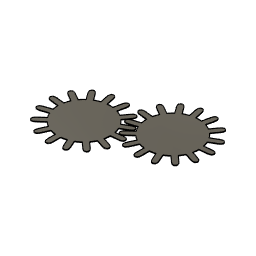
Gears (Autodesk Fusion 360 design; units mm, degrees)
Autodesk Fusion 360 part; units mm, degrees
sketch "Sketch1" plane through (0, 0, 0) normal (0, 0, 1) x (1, 0, 0)
  line L0 (-5, -63.7603) -> (-5, -49.7494)
  spline S0 degree 5 poles (-5, -63.7603) (-5, -64.7116) (-4.9363, -66.4553) (-4.6499, -68.5942) (-3.9278, -70.5592) (-2.6801, -71.8795) (-1.3088, -72.4515) (0, -72.5944) (1.3088, -72.4515) (2.68, -71.8795) (3.9278, -70.5592) (4.6499, -68.5942) (4.9363, -66.4553) (5, -64.7116) (5, -63.7603) knots 0 0 0 0 0 0 0.1 0.2 0.3 0.4 0.5 0.6 0.7 0.8 0.9 1 1 1 1 1 1
  line L1 (-5, -60.7603) -> (-5, -66.7603)
  line L2 (5, -66.7603) -> (5, -60.7603)
  line L3 (-0.7054, -72.5206) -> (0.7054, -72.5206)
  spline S1 degree 5 poles (21.3659, -60.2816) (21.7529, -61.1507) (22.5203, -62.7177) (23.6519, -64.5552) (25.1108, -66.0566) (26.7877, -66.7553) (28.2731, -66.7201) (29.5268, -66.3183) (30.6643, -65.6554) (31.6844, -64.5751) (32.2872, -62.8615) (32.1477, -60.7726) (31.5394, -58.7022) (30.8883, -57.0833) (30.5014, -56.2142) knots 0 0 0 0 0 0 0.1 0.2 0.3 0.4 0.5 0.6 0.7 0.8 0.9 1 1 1 1 1 1
  line L4 (44.0375, -46.3797) -> (33.6253, -37.0046)
  spline S2 degree 5 poles (44.0375, -46.3797) (44.7444, -47.0162) (46.0829, -48.1357) (47.864, -49.354) (49.8075, -50.1322) (51.6236, -50.0885) (52.9662, -49.4522) (53.9482, -48.5752) (54.7177, -47.5069) (55.2102, -46.1051) (55.0639, -44.2944) (54.0868, -42.4429) (52.689, -40.7989) (51.4357, -39.5848) (50.7288, -38.9482) knots 0 0 0 0 0 0 0.1 0.2 0.3 0.4 0.5 0.6 0.7 0.8 0.9 1 1 1 1 1 1
  spline S3 degree 5 poles (59.0946, -24.4583) (59.9993, -24.7523) (61.6773, -25.2305) (63.8, -25.6191) (65.892, -25.5396) (67.5333, -24.7609) (68.5011, -23.6335) (69.0414, -22.4329) (69.3099, -21.144) (69.1897, -19.6631) (68.3195, -18.0684) (66.6739, -16.7744) (64.7282, -15.8411) (63.0895, -15.2417) (62.1847, -14.9477) knots 0 0 0 0 0 0 0.1 0.2 0.3 0.4 0.5 0.6 0.7 0.8 0.9 1 1 1 1 1 1
  line L5 (63.9337, 1.6922) -> (49.9995, 0.2276)
  spline S4 degree 5 poles (63.9337, 1.6922) (64.8797, 1.7916) (66.6072, 2.0372) (68.7045, 2.5456) (70.5832, 3.4692) (71.7659, 4.8481) (72.1914, 6.2716) (72.1968, 7.5882) (71.9178, 8.8749) (71.2056, 10.1788) (69.7621, 11.2817) (67.7324, 11.7945) (65.5753, 11.8557) (63.8345, 11.7368) (62.8884, 11.6374) knots 0 0 0 0 0 0 0.1 0.2 0.3 0.4 0.5 0.6 0.7 0.8 0.9 1 1 1 1 1 1
  line L6 (57.718, 27.55) -> (45.5842, 20.5446)
  spline S5 degree 5 poles (57.718, 27.55) (58.5419, 28.0257) (60.0201, 28.9527) (61.7293, 30.2701) (63.07, 31.878) (63.5895, 33.6188) (63.3993, 35.0923) (62.8686, 36.2972) (62.0905, 37.3592) (60.9095, 38.2608) (59.1422, 38.6812) (57.0793, 38.324) (55.0838, 37.5026) (53.5419, 36.6859) (52.718, 36.2103) knots 0 0 0 0 0 0 0.1 0.2 0.3 0.4 0.5 0.6 0.7 0.8 0.9 1 1 1 1 1 1
  spline S6 degree 5 poles (41.5224, 48.6442) (42.0816, 49.4139) (43.055, 50.862) (44.0805, 52.7607) (44.6513, 54.7749) (44.4179, 56.5765) (43.6448, 57.8452) (42.6699, 58.7301) (41.5271, 59.3838) (40.0815, 59.7271) (38.296, 59.3923) (36.5568, 58.227) (35.0679, 56.665) (33.9914, 55.2917) (33.4323, 54.5221) knots 0 0 0 0 0 0 0.1 0.2 0.3 0.4 0.5 0.6 0.7 0.8 0.9 1 1 1 1 1 1
  spline S7 degree 5 poles (18.1472, 61.3274) (18.345, 62.2579) (18.6453, 63.9768) (18.8098, 66.1285) (18.5121, 68.2007) (17.5661, 69.7516) (16.3437, 70.5962) (15.0932, 71.0081) (13.7833, 71.1404) (12.3231, 70.866) (10.8281, 69.8339) (9.7132, 68.062) (8.9884, 66.0294) (8.5636, 64.3371) (8.3658, 63.4065) knots 0 0 0 0 0 0 0.1 0.2 0.3 0.4 0.5 0.6 0.7 0.8 0.9 1 1 1 1 1 1
  spline S8 degree 5 poles (-8.3658, 63.4065) (-8.5636, 64.3371) (-8.9884, 66.0294) (-9.7132, 68.062) (-10.8281, 69.8339) (-12.3231, 70.866) (-13.7833, 71.1404) (-15.0932, 71.0081) (-16.3437, 70.5962) (-17.5661, 69.7516) (-18.512, 68.2007) (-18.8098, 66.1285) (-18.6453, 63.9768) (-18.345, 62.2579) (-18.1472, 61.3274) knots 0 0 0 0 0 0 0.1 0.2 0.3 0.4 0.5 0.6 0.7 0.8 0.9 1 1 1 1 1 1
  spline S9 degree 5 poles (-33.4323, 54.5221) (-33.9914, 55.2917) (-35.0679, 56.665) (-36.5568, 58.227) (-38.296, 59.3923) (-40.0815, 59.7271) (-41.5271, 59.3838) (-42.6699, 58.7301) (-43.6448, 57.8452) (-44.4179, 56.5765) (-44.6513, 54.7749) (-44.0805, 52.7607) (-43.055, 50.862) (-42.0816, 49.4139) (-41.5224, 48.6442) knots 0 0 0 0 0 0 0.1 0.2 0.3 0.4 0.5 0.6 0.7 0.8 0.9 1 1 1 1 1 1
  spline S10 degree 5 poles (-52.718, 36.2103) (-53.5419, 36.6859) (-55.0838, 37.5026) (-57.0793, 38.324) (-59.1422, 38.6812) (-60.9095, 38.2608) (-62.0905, 37.3592) (-62.8686, 36.2972) (-63.3993, 35.0923) (-63.5895, 33.6188) (-63.07, 31.878) (-61.7293, 30.2701) (-60.0201, 28.9527) (-58.5419, 28.0257) (-57.718, 27.55) knots 0 0 0 0 0 0 0.1 0.2 0.3 0.4 0.5 0.6 0.7 0.8 0.9 1 1 1 1 1 1
  spline S11 degree 5 poles (-62.8884, 11.6374) (-63.8345, 11.7368) (-65.5753, 11.8557) (-67.7324, 11.7945) (-69.7621, 11.2817) (-71.2056, 10.1788) (-71.9178, 8.8749) (-72.1968, 7.5882) (-72.1914, 6.2716) (-71.7659, 4.8481) (-70.5832, 3.4692) (-68.7045, 2.5456) (-66.6072, 2.0372) (-64.8797, 1.7916) (-63.9337, 1.6922) knots 0 0 0 0 0 0 0.1 0.2 0.3 0.4 0.5 0.6 0.7 0.8 0.9 1 1 1 1 1 1
  spline S12 degree 5 poles (-62.1847, -14.9477) (-63.0895, -15.2417) (-64.7282, -15.8411) (-66.6739, -16.7744) (-68.3195, -18.0684) (-69.1897, -19.6631) (-69.3099, -21.144) (-69.0414, -22.4329) (-68.5011, -23.6335) (-67.5333, -24.7609) (-65.892, -25.5395) (-63.8, -25.6191) (-61.6773, -25.2305) (-59.9993, -24.7523) (-59.0946, -24.4583) knots 0 0 0 0 0 0 0.1 0.2 0.3 0.4 0.5 0.6 0.7 0.8 0.9 1 1 1 1 1 1
  spline S13 degree 5 poles (-50.7288, -38.9482) (-51.4357, -39.5848) (-52.689, -40.7989) (-54.0868, -42.4429) (-55.0639, -44.2944) (-55.2102, -46.1051) (-54.7177, -47.5069) (-53.9482, -48.5752) (-52.9662, -49.4522) (-51.6236, -50.0885) (-49.8075, -50.1322) (-47.864, -49.354) (-46.0829, -48.1357) (-44.7444, -47.0162) (-44.0375, -46.3797) knots 0 0 0 0 0 0 0.1 0.2 0.3 0.4 0.5 0.6 0.7 0.8 0.9 1 1 1 1 1 1
  spline S14 degree 5 poles (-30.5014, -56.2142) (-30.8883, -57.0833) (-31.5394, -58.7022) (-32.1477, -60.7726) (-32.2872, -62.8614) (-31.6844, -64.5751) (-30.6643, -65.6554) (-29.5268, -66.3183) (-28.2731, -66.7201) (-26.7877, -66.7553) (-25.1108, -66.0566) (-23.6519, -64.5552) (-22.5203, -62.7177) (-21.7529, -61.1507) (-21.3659, -60.2816) knots 0 0 0 0 0 0 0.1 0.2 0.3 0.4 0.5 0.6 0.7 0.8 0.9 1 1 1 1 1 1
  line L7 (18.1472, 61.3274) -> (15.2342, 47.6227)
  line L8 (5.4527, 49.7018) -> (8.3658, 63.4065)
  line L9 (-8.3658, 63.4065) -> (-5.4527, 49.7018)
  line L10 (-15.2342, 47.6227) -> (-18.1472, 61.3274)
  line L11 (-33.4323, 54.5221) -> (-25.1969, 43.187)
  line L12 (-33.287, 37.3092) -> (-41.5224, 48.6442)
  line L13 (-52.718, 36.2103) -> (-40.5842, 29.2048)
  line L14 (-45.5842, 20.5446) -> (-57.718, 27.55)
  line L15 (-62.8884, 11.6374) -> (-48.9542, 10.1728)
  line L16 (-49.9995, 0.2276) -> (-63.9337, 1.6922)
  line L17 (-62.1847, -14.9477) -> (-48.8595, -10.6181)
  line L18 (-45.7694, -20.1287) -> (-59.0946, -24.4583)
  line L19 (-50.7288, -38.9482) -> (-40.3166, -29.5731)
  line L20 (-33.6253, -37.0046) -> (-44.0375, -46.3797)
  line L21 (-30.5014, -56.2142) -> (-24.8026, -43.4146)
  line L22 (-15.6672, -47.482) -> (-21.3659, -60.2816)
  line L23 (5, -49.7494) -> (5, -63.7603)
  line L24 (21.3659, -60.2816) -> (15.6672, -47.482)
  line L25 (24.8026, -43.4146) -> (30.5014, -56.2142)
  line L26 (40.3166, -29.5731) -> (50.7288, -38.9482)
  line L27 (59.0946, -24.4583) -> (45.7694, -20.1287)
  line L28 (48.8595, -10.6181) -> (62.1847, -14.9477)
  line L29 (48.9542, 10.1728) -> (62.8884, 11.6374)
  line L30 (40.5842, 29.2048) -> (52.718, 36.2103)
  line L31 (25.1969, 43.187) -> (33.4323, 54.5221)
  line L32 (41.5224, 48.6442) -> (33.287, 37.3092)
  arc A0 (25.1969, 43.187) -> (15.2342, 47.6227) centre (0, 0) ccw
  arc A1 (5.4527, 49.7018) -> (-5.4527, 49.7018) centre (0, 0) ccw
  arc A2 (-15.2342, 47.6227) -> (-25.1969, 43.187) centre (0, 0) ccw
  arc A3 (-33.287, 37.3092) -> (-40.5842, 29.2048) centre (0, 0) ccw
  arc A4 (-45.5842, 20.5446) -> (-48.9542, 10.1728) centre (0, 0) ccw
  arc A5 (-49.9995, 0.2276) -> (-48.8595, -10.6181) centre (0, 0) ccw
  arc A6 (-45.7694, -20.1287) -> (-40.3166, -29.5731) centre (0, 0) ccw
  arc A7 (-33.6253, -37.0046) -> (-24.8026, -43.4146) centre (0, 0) ccw
  arc A8 (-15.6672, -47.482) -> (-5, -49.7494) centre (0, 0) ccw
  arc A9 (5, -49.7494) -> (15.6672, -47.482) centre (0, 0) ccw
  arc A10 (24.8026, -43.4146) -> (33.6253, -37.0046) centre (0, 0) ccw
  arc A11 (40.3166, -29.5731) -> (45.7694, -20.1287) centre (0, 0) ccw
  arc A12 (48.8595, -10.6181) -> (49.9995, 0.2276) centre (0, 0) ccw
  arc A13 (48.9542, 10.1728) -> (45.5842, 20.5446) centre (0, 0) ccw
  arc A14 (40.5842, 29.2048) -> (33.287, 37.3092) centre (0, 0) ccw
  line L33 (-245, -49.7494) -> (-245, -63.7603)
  line L34 (-255, -63.7603) -> (-255, -49.7494)
  spline S15 degree 5 poles (-255, -63.7603) (-255, -64.7116) (-254.9363, -66.4553) (-254.6499, -68.5942) (-253.9278, -70.5592) (-252.6801, -71.8795) (-251.3088, -72.4515) (-250, -72.5944) (-248.6912, -72.4515) (-247.32, -71.8795) (-246.0722, -70.5592) (-245.3501, -68.5942) (-245.0637, -66.4553) (-245, -64.7116) (-245, -63.7603) knots 0 0 0 0 0 0 0.1 0.2 0.3 0.4 0.5 0.6 0.7 0.8 0.9 1 1 1 1 1 1
  line L35 (-255, -60.7603) -> (-255, -66.7603)
  line L36 (-250.7054, -72.5206) -> (-249.2946, -72.5206)
  line L37 (-245, -66.7603) -> (-245, -60.7603)
  line L38 (-225.1974, -43.4146) -> (-219.4986, -56.2142)
  line L39 (-228.6341, -60.2816) -> (-234.3328, -47.482)
  spline S16 degree 5 poles (-228.6341, -60.2816) (-228.2471, -61.1507) (-227.4797, -62.7177) (-226.3481, -64.5552) (-224.8892, -66.0566) (-223.2123, -66.7553) (-221.7269, -66.7201) (-220.4732, -66.3183) (-219.3357, -65.6554) (-218.3156, -64.5751) (-217.7128, -62.8615) (-217.8523, -60.7726) (-218.4606, -58.7022) (-219.1117, -57.0833) (-219.4986, -56.2142) knots 0 0 0 0 0 0 0.1 0.2 0.3 0.4 0.5 0.6 0.7 0.8 0.9 1 1 1 1 1 1
  line L40 (-209.6834, -29.5731) -> (-199.2712, -38.9482)
  line L41 (-205.9625, -46.3797) -> (-216.3747, -37.0046)
  spline S17 degree 5 poles (-205.9625, -46.3797) (-205.2556, -47.0162) (-203.9171, -48.1357) (-202.136, -49.354) (-200.1925, -50.1322) (-198.3764, -50.0885) (-197.0338, -49.4522) (-196.0518, -48.5752) (-195.2823, -47.5069) (-194.7898, -46.1051) (-194.9361, -44.2944) (-195.9132, -42.4429) (-197.311, -40.7989) (-198.5643, -39.5848) (-199.2712, -38.9482) knots 0 0 0 0 0 0 0.1 0.2 0.3 0.4 0.5 0.6 0.7 0.8 0.9 1 1 1 1 1 1
  line L42 (-201.1405, -10.6181) -> (-187.8153, -14.9477)
  line L43 (-190.9054, -24.4583) -> (-204.2306, -20.1287)
  spline S18 degree 5 poles (-190.9054, -24.4583) (-190.0007, -24.7523) (-188.3227, -25.2305) (-186.2, -25.6191) (-184.108, -25.5396) (-182.4667, -24.7609) (-181.4989, -23.6335) (-180.9586, -22.4329) (-180.6901, -21.144) (-180.8103, -19.6631) (-181.6805, -18.0684) (-183.3261, -16.7744) (-185.2718, -15.8411) (-186.9105, -15.2417) (-187.8153, -14.9477) knots 0 0 0 0 0 0 0.1 0.2 0.3 0.4 0.5 0.6 0.7 0.8 0.9 1 1 1 1 1 1
  line L44 (-201.0458, 10.1728) -> (-187.1116, 11.6374)
  line L45 (-186.0663, 1.6922) -> (-200.0005, 0.2276)
  spline S19 degree 5 poles (-186.0663, 1.6922) (-185.1203, 1.7916) (-183.3928, 2.0372) (-181.2955, 2.5456) (-179.4168, 3.4692) (-178.2341, 4.8481) (-177.8086, 6.2716) (-177.8032, 7.5882) (-178.0822, 8.8749) (-178.7944, 10.1788) (-180.2379, 11.2817) (-182.2676, 11.7945) (-184.4247, 11.8557) (-186.1655, 11.7368) (-187.1116, 11.6374) knots 0 0 0 0 0 0 0.1 0.2 0.3 0.4 0.5 0.6 0.7 0.8 0.9 1 1 1 1 1 1
  line L46 (-209.4158, 29.2048) -> (-197.282, 36.2103)
  line L47 (-192.282, 27.55) -> (-204.4158, 20.5446)
  spline S20 degree 5 poles (-192.282, 27.55) (-191.4581, 28.0257) (-189.9799, 28.9527) (-188.2707, 30.2701) (-186.93, 31.878) (-186.4105, 33.6188) (-186.6007, 35.0923) (-187.1314, 36.2972) (-187.9095, 37.3592) (-189.0905, 38.2608) (-190.8578, 38.6812) (-192.9207, 38.324) (-194.9162, 37.5026) (-196.4581, 36.6859) (-197.282, 36.2103) knots 0 0 0 0 0 0 0.1 0.2 0.3 0.4 0.5 0.6 0.7 0.8 0.9 1 1 1 1 1 1
  line L48 (-224.8031, 43.187) -> (-216.5677, 54.5221)
  line L49 (-208.4776, 48.6442) -> (-216.713, 37.3092)
  spline S21 degree 5 poles (-208.4776, 48.6442) (-207.9184, 49.4139) (-206.945, 50.862) (-205.9195, 52.7607) (-205.3487, 54.7749) (-205.5821, 56.5765) (-206.3552, 57.8452) (-207.3301, 58.7301) (-208.4729, 59.3838) (-209.9185, 59.7271) (-211.704, 59.3923) (-213.4432, 58.227) (-214.9321, 56.665) (-216.0086, 55.2917) (-216.5677, 54.5221) knots 0 0 0 0 0 0 0.1 0.2 0.3 0.4 0.5 0.6 0.7 0.8 0.9 1 1 1 1 1 1
  line L50 (-244.5473, 49.7018) -> (-241.6342, 63.4065)
  line L51 (-231.8528, 61.3274) -> (-234.7658, 47.6227)
  spline S22 degree 5 poles (-231.8528, 61.3274) (-231.655, 62.2579) (-231.3547, 63.9768) (-231.1902, 66.1285) (-231.4879, 68.2007) (-232.4339, 69.7516) (-233.6563, 70.5962) (-234.9068, 71.0081) (-236.2167, 71.1404) (-237.6769, 70.866) (-239.1719, 69.8339) (-240.2868, 68.062) (-241.0116, 66.0294) (-241.4364, 64.3371) (-241.6342, 63.4065) knots 0 0 0 0 0 0 0.1 0.2 0.3 0.4 0.5 0.6 0.7 0.8 0.9 1 1 1 1 1 1
  line L52 (-265.2342, 47.6227) -> (-268.1472, 61.3274)
  line L53 (-258.3658, 63.4065) -> (-255.4527, 49.7018)
  spline S23 degree 5 poles (-258.3658, 63.4065) (-258.5636, 64.3371) (-258.9884, 66.0294) (-259.7132, 68.062) (-260.8281, 69.8339) (-262.3231, 70.866) (-263.7833, 71.1404) (-265.0932, 71.0081) (-266.3437, 70.5962) (-267.5661, 69.7516) (-268.512, 68.2007) (-268.8098, 66.1285) (-268.6453, 63.9768) (-268.345, 62.2579) (-268.1472, 61.3274) knots 0 0 0 0 0 0 0.1 0.2 0.3 0.4 0.5 0.6 0.7 0.8 0.9 1 1 1 1 1 1
  line L54 (-283.287, 37.3092) -> (-291.5224, 48.6442)
  line L55 (-283.4323, 54.5221) -> (-275.1969, 43.187)
  spline S24 degree 5 poles (-283.4323, 54.5221) (-283.9914, 55.2917) (-285.0679, 56.665) (-286.5568, 58.227) (-288.296, 59.3923) (-290.0815, 59.7271) (-291.5271, 59.3838) (-292.6699, 58.7301) (-293.6448, 57.8452) (-294.4179, 56.5765) (-294.6513, 54.7749) (-294.0805, 52.7607) (-293.055, 50.862) (-292.0816, 49.4139) (-291.5224, 48.6442) knots 0 0 0 0 0 0 0.1 0.2 0.3 0.4 0.5 0.6 0.7 0.8 0.9 1 1 1 1 1 1
  line L56 (-295.5842, 20.5446) -> (-307.718, 27.55)
  line L57 (-302.718, 36.2103) -> (-290.5842, 29.2048)
  spline S25 degree 5 poles (-302.718, 36.2103) (-303.5419, 36.6859) (-305.0838, 37.5026) (-307.0793, 38.324) (-309.1422, 38.6812) (-310.9095, 38.2608) (-312.0905, 37.3592) (-312.8686, 36.2972) (-313.3993, 35.0923) (-313.5895, 33.6188) (-313.07, 31.878) (-311.7293, 30.2701) (-310.0201, 28.9527) (-308.5419, 28.0257) (-307.718, 27.55) knots 0 0 0 0 0 0 0.1 0.2 0.3 0.4 0.5 0.6 0.7 0.8 0.9 1 1 1 1 1 1
  line L58 (-299.9995, 0.2276) -> (-313.9337, 1.6922)
  line L59 (-312.8884, 11.6374) -> (-298.9542, 10.1728)
  spline S26 degree 5 poles (-312.8884, 11.6374) (-313.8345, 11.7368) (-315.5753, 11.8557) (-317.7324, 11.7945) (-319.7621, 11.2817) (-321.2056, 10.1788) (-321.9178, 8.8749) (-322.1968, 7.5882) (-322.1914, 6.2716) (-321.7659, 4.8481) (-320.5832, 3.4692) (-318.7045, 2.5456) (-316.6072, 2.0372) (-314.8797, 1.7916) (-313.9337, 1.6922) knots 0 0 0 0 0 0 0.1 0.2 0.3 0.4 0.5 0.6 0.7 0.8 0.9 1 1 1 1 1 1
  line L60 (-295.7694, -20.1287) -> (-309.0946, -24.4583)
  line L61 (-312.1847, -14.9477) -> (-298.8595, -10.6181)
  spline S27 degree 5 poles (-312.1847, -14.9477) (-313.0895, -15.2417) (-314.7282, -15.8411) (-316.6739, -16.7744) (-318.3195, -18.0684) (-319.1897, -19.6631) (-319.3099, -21.144) (-319.0414, -22.4329) (-318.5011, -23.6335) (-317.5333, -24.7609) (-315.892, -25.5395) (-313.8, -25.6191) (-311.6773, -25.2305) (-309.9993, -24.7523) (-309.0946, -24.4583) knots 0 0 0 0 0 0 0.1 0.2 0.3 0.4 0.5 0.6 0.7 0.8 0.9 1 1 1 1 1 1
  line L62 (-283.6253, -37.0046) -> (-294.0375, -46.3797)
  line L63 (-300.7288, -38.9482) -> (-290.3166, -29.5731)
  spline S28 degree 5 poles (-300.7288, -38.9482) (-301.4357, -39.5848) (-302.689, -40.7989) (-304.0868, -42.4429) (-305.0639, -44.2944) (-305.2102, -46.1051) (-304.7177, -47.5069) (-303.9482, -48.5752) (-302.9662, -49.4522) (-301.6236, -50.0885) (-299.8075, -50.1322) (-297.864, -49.354) (-296.0829, -48.1357) (-294.7444, -47.0162) (-294.0375, -46.3797) knots 0 0 0 0 0 0 0.1 0.2 0.3 0.4 0.5 0.6 0.7 0.8 0.9 1 1 1 1 1 1
  line L64 (-265.6672, -47.482) -> (-271.3659, -60.2816)
  line L65 (-280.5014, -56.2142) -> (-274.8026, -43.4146)
  spline S29 degree 5 poles (-280.5014, -56.2142) (-280.8883, -57.0833) (-281.5394, -58.7022) (-282.1477, -60.7726) (-282.2872, -62.8614) (-281.6844, -64.5751) (-280.6643, -65.6554) (-279.5268, -66.3183) (-278.2731, -66.7201) (-276.7877, -66.7553) (-275.1108, -66.0566) (-273.6519, -64.5552) (-272.5203, -62.7177) (-271.7529, -61.1507) (-271.3659, -60.2816) knots 0 0 0 0 0 0 0.1 0.2 0.3 0.4 0.5 0.6 0.7 0.8 0.9 1 1 1 1 1 1
  arc A15 (-265.2342, 47.6227) -> (-275.1969, 43.187) centre (-250, 0) ccw
  arc A16 (-283.287, 37.3092) -> (-290.5842, 29.2048) centre (-250, 0) ccw
  arc A17 (-295.5842, 20.5446) -> (-298.9542, 10.1728) centre (-250, 0) ccw
  arc A18 (-299.9995, 0.2276) -> (-298.8595, -10.6181) centre (-250, 0) ccw
  arc A19 (-295.7694, -20.1287) -> (-290.3166, -29.5731) centre (-250, 0) ccw
  arc A20 (-283.6253, -37.0046) -> (-274.8026, -43.4146) centre (-250, 0) ccw
  arc A21 (-265.6672, -47.482) -> (-255, -49.7494) centre (-250, 0) ccw
  arc A22 (-245, -49.7494) -> (-234.3328, -47.482) centre (-250, 0) ccw
  arc A23 (-225.1974, -43.4146) -> (-216.3747, -37.0046) centre (-250, 0) ccw
  arc A24 (-209.6834, -29.5731) -> (-204.2306, -20.1287) centre (-250, 0) ccw
  arc A25 (-201.1405, -10.6181) -> (-200.0005, 0.2276) centre (-250, 0) ccw
  arc A26 (-201.0458, 10.1728) -> (-204.4158, 20.5446) centre (-250, 0) ccw
  arc A27 (-209.4158, 29.2048) -> (-216.713, 37.3092) centre (-250, 0) ccw
  arc A28 (-224.8031, 43.187) -> (-234.7658, 47.6227) centre (-250, 0) ccw
  arc A29 (-244.5473, 49.7018) -> (-255.4527, 49.7018) centre (-250, 0) ccw
  point P0 (0, -72.5206)
  point P1 (29.4968, -66.2509)
  point P2 (53.8933, -48.5258)
  point P3 (68.9712, -22.4101)
  point P4 (72.1233, 7.5805)
  point P5 (62.8047, 36.2603)
  point P6 (42.6265, 58.6704)
  point P7 (15.0779, 70.9358)
  point P8 (-15.0779, 70.9358)
  point P9 (-42.6265, 58.6704)
  point P10 (-62.8047, 36.2603)
  point P11 (-72.1233, 7.5805)
  point P12 (-68.9712, -22.4101)
  point P13 (-53.8933, -48.5258)
  point P14 (-29.4968, -66.2509)
  point P15 (-250, -72.5206)
  point P16 (-220.5032, -66.2509)
  point P17 (-196.1067, -48.5258)
  point P18 (-181.0288, -22.4101)
  point P19 (-177.8767, 7.5805)
  point P20 (-187.1953, 36.2603)
  point P21 (-207.3735, 58.6704)
  point P22 (-234.9221, 70.9358)
  point P23 (-265.0779, 70.9358)
  point P24 (-292.6265, 58.6704)
  point P25 (-312.8047, 36.2603)
  point P26 (-322.1233, 7.5805)
  point P27 (-318.9712, -22.4101)
  point P28 (-303.8933, -48.5258)
  point P29 (-279.4968, -66.2509)
  dimension "d8" = 10
  dimension "d9" = 10.9055
  dimension "d10" = 14.0109
  dimension "d11" = 14.0109
  dimension "d20" = 360
  constraint coincident A0.centre A1.centre
  constraint midpoint L0.start L1
  constraint midpoint S0.end L2
  constraint midpoint P0 L3
  constraint coincident L8.start A0
  constraint coincident L9.end A0
  constraint coincident L10.start A0
  constraint coincident L11.end A0
  constraint coincident L12.start A0
  constraint coincident L13.end A0
  constraint coincident L14.start A0
  constraint coincident L15.end A0
  constraint coincident L16.start A0
  constraint coincident L17.end A0
  constraint coincident L18.start A0
  constraint coincident L19.end A0
  constraint coincident L20.start A0
  constraint coincident L21.end A0
  constraint coincident L22.start A0
  constraint coincident L23.start A0
  constraint coincident L24.end A0
  constraint coincident L25.start A0
  constraint coincident L26.start A0
  constraint coincident L27.end A0
  constraint coincident L28.start A0
  constraint coincident L29.start A0
  constraint coincident L30.start A0
  constraint coincident L5.end A0
  constraint coincident L4.end A0
  constraint coincident L6.end A0
  constraint coincident L0.end A0
  constraint concentric A0 A1
  constraint concentric A1 A2
  constraint concentric A2 A3
  constraint concentric A3 A4
  constraint concentric A4 A5
  constraint concentric A5 A6
  constraint concentric A6 A7
  constraint concentric A7 A8
  constraint concentric A8 A9
  constraint concentric A9 A10
  constraint concentric A10 A11
  constraint concentric A11 A12
  constraint concentric A12 A13
  constraint concentric A13 A14
  constraint midpoint L34.start L35
  constraint midpoint L33.end L37
  constraint midpoint P15 L36
  constraint concentric A15 A22
  constraint concentric A15 A16
  constraint concentric A16 A17
  constraint concentric A17 A18
  constraint concentric A18 A19
  constraint concentric A19 A20
  constraint concentric A20 A21
  constraint concentric A22 A23
  constraint concentric A23 A24
  constraint concentric A24 A25
  constraint concentric A25 A26
  constraint concentric A26 A27
  constraint concentric A27 A28
  constraint concentric A28 A29
  measures "d8" distance of L9 L10
  measures "d9" distance of L10.start L11.end
  measures "d10" distance of S7.end L8.start
  measures "d11" distance of S9.end L12.start
extrude "Extrude1" add sketch "Sketch1" along normal blind 1 contours L0 S0 L1 L2 S1 L4 S2 S3 L5 S4 L6 S5 S6 S7 S8 S9 S10 S11 S12 S13 S14 L7 L8 L9 L10 L11 L12 L13 L14 L15 L16 L17 L18 L19 L20 L21 L22 L23 L24 L25 L26 L27 L28 L29 L30 L31 L32 A0 A1 A2 A3 A4 A5 A6 A7 A8 A9 A10 A11 A12 A13 A14 makes body 1
copy_body "CopyPasteBodies2" bodies 1 makes body 2
move_body "Move1" bodies 2 to x (1, 0, 0) y (0, 1, 0) z (0, 0, 1) at (-130, 0, 0)
move_body "Move2" bodies 2 to x (1, 0, 0) y (0, 1, 0) z (0, 0, 1) at (22.3281, -62.2468, 0)
copy_body "Body->Comp1" bodies 2 removing the originals makes body 3 in component "Component"
copy_body "Body->Comp2" bodies 1 removing the originals makes body 4 in component "Component'"
component "Component" placed x (1, 0, 0) y (0, 1, 0) z (0, 0, 1) at (0, 0, 0)
component "Component'" placed x (1, 0, 0) y (0, 1, 0) z (0, 0, 1) at (0, 0, 0)
